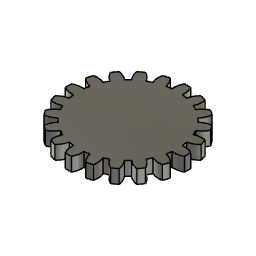
Spur Gear (Autodesk Fusion 360 design; units mm, degrees)
Autodesk Fusion 360 part; units mm, degrees
sketch "Spur Gear" plane through (0, 0, 0) normal (0, 0, 1) x (1, 0, 0)
  line L0 (0, 0) -> (1.1341, 7.1607)
  arc A0 (0.7578, 7.2103) -> (0.4579, 8.738) centre (-1.8742, 7.4869) ccw
  arc A1 (0.4579, 8.738) -> (0, 8.75) centre (0, 0) ccw
  arc A2 (1.1341, 7.1607) -> (0.7578, 7.2103) centre (0, 0) ccw
  arc A3 (-0.4579, 8.738) -> (-0.7578, 7.2103) centre (1.8742, 7.4869) ccw
  arc A4 (0, 8.75) -> (-0.4579, 8.738) centre (0, 0) ccw
  arc A5 (-0.7578, 7.2103) -> (-1.1341, 7.1607) centre (0, 0) ccw
  line L1 (0, 0) -> (-1.1341, 7.1607)
  constraint coincident L0.start A1.centre
extrude "Extrude1" add sketch "Spur Gear" along normal blind 2 makes body 1
pattern_circular "C-Pattern1" count 20 over 360 about axis through (0, 0, 1.75) along (0, 0, 1) of bodies 1 makes body 2 at (-0.378, 2.3869, 0.6667) makes body 3 at (-2.8254, 3.8888, 0) makes body 4 at (-3.8888, 2.8254, 0) makes body 5 at (-4.5716, 1.4854, 0) makes body 6 at (-4.8069, 0, 0) makes body 7 at (-4.5716, -1.4854, 0) makes body 8 at (-3.8888, -2.8254, 0) makes body 9 at (-2.8254, -3.8888, 0) makes body 10 at (-1.4854, -4.5716, 0) makes body 11 at (0, -4.8069, 0) makes body 12 at (1.4854, -4.5716, 0) makes body 13 at (2.8254, -3.8888, 0) makes body 14 at (3.8888, -2.8254, 0) makes body 15 at (4.5716, -1.4854, 0) makes body 16 at (4.8069, 0, 0) makes body 17 at (4.5716, 1.4854, 0) makes body 18 at (3.8888, 2.8254, 0) makes body 19 at (2.8254, 3.8888, 0) makes body 20 at (0.378, 2.3869, 1.3333)
combine "Combine1" operation add target body 17 tool bodies 14 10 18 5 2 4 7 19 9 8 15 16 1 20 3 12 13 6 11
named bodies: "Spur Gear"
